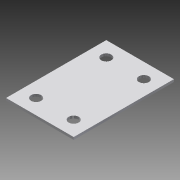
# Autodesk Inventor part: BracketHalf
Saved by Autodesk Inventor 2014 SP1 (Build 180222100, 222)
## iProperties
Created: 2015-03-22
Part Number: BracketHalf
Material: Generic
Document SubType Name: Sheet Metal
Designer: david
Density: 1 g/cm^3
Sheet Metal Rule: Default
Appearance: Default
Author: david
Autodesk Inventor part; units mm, degrees
ref_plane "YZ Plane" through (0, 0, 0) normal (1, 0, 0) x (0, 1, 0)
ref_plane "XZ Plane" through (0, 0, 0) normal (0, 1, 0) x (-1, 0, 0)
ref_plane "XY Plane" through (0, 0, 0) normal (0, 0, 1) x (1, 0, 0)
sketch "Sketch1" plane through (0, 0, 0) normal (0, 1, 0) x (-1, 0, 0)
  line L0 (-27, 20) -> (0, 20)
  line L1 (0, 20) -> (0, 0) construction
  line L2 (0, 0) -> (-27, 0) construction
  line L3 (-27, 0) -> (-27, 20)
  line L4 (-37.8717, 14) -> (4.6091, 14) construction
  circle A0 centre (-6, 14) radius 2
  circle A1 centre (-21, 14) radius 2
  line L5 (-27, -20) -> (0, -20)
  line L6 (0, -20) -> (0, 0) construction
  line L7 (-27, 0) -> (-27, -20)
  line L8 (-37.8717, -14) -> (4.6091, -14) construction
  circle A2 centre (-6, -14) radius 2
  circle A3 centre (-21, -14) radius 2
  line L9 (0, 20) -> (0, -20)
  dimension "d1" = 20
  dimension "d2" = 6
  dimension "d3" = 4
  dimension "d4" = 6
  dimension "d5" = 21
  dimension "d7" = 6
  measures "d1" distance of L2.end L0.start
  measures "d2" distance between parallel lines of L0 L4
  measures "d3" diameter of A1
  measures "d4" distance from line of L3 A1.centre
  measures "d5" distance from line of L3 A0.centre
  measures "d7" distance from line of L1 A0.centre
extrude "Plate1" add sketch "Sketch1" along normal blind 1
equation "\"BendRadius\" = Thickness"
equation "\"BendReliefWidth\" = Thickness"
equation "\"BendReliefDepth\" = 0.5 * Thickness"
equation "\"CornerReliefSize\" = 4 * Thickness"
equation "\"MinimumRemnant\" = 2 * Thickness"
equation "\"TransitionRadius\" = BendRadius"
equation "\"JacobiRadiusSize\" = BendRadius"
equation "\"GapSize\" = Thickness"
equation "\"d6\" = BendRadius"
equation "\"Thickness\" = 1"
body "Solid1"
